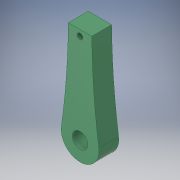
# Autodesk Inventor part: joint3_rot
Saved by Autodesk Inventor 2019 (Build 230136000, 136)
## iProperties
Created: 2019-12-29
Part Number: joint3_rot
Material: Пластик АБС
Document SubType Name: Modeling
Designer: Петров Иван
Density: 1.06 g/cm^3
Appearance: Гладкий — темный цвет морской волны
Author: Петров Иван
Autodesk Inventor part; units mm, degrees
ref_plane "YZ Plane" through (0, 0, 0) normal (1, 0, 0) x (0, 1, 0)
ref_plane "XZ Plane" through (0, 0, 0) normal (0, 1, 0) x (-1, 0, 0)
ref_plane "XY Plane" through (0, 0, 0) normal (0, 0, 1) x (1, 0, 0)
sketch "Эскиз1" plane through (0, 0, 0) normal (0, 0, 1) x (1, 0, 0)
  circle A0 centre (0, 0) radius 3.9
  line L0 (-3.9, 0) -> (-3.9, 42.3207)
  line L1 (3.9, 42.3207) -> (3.9, 0)
  arc A1 (3.9, 42.3207) -> (-3.9, 42.3207) centre (0, 0) ccw
  line L2 (-3.9, 42.3207) -> (-3.9, 48.3207)
  line L3 (-3.9, 48.3207) -> (3.9, 48.3207)
  line L4 (3.9, 48.3207) -> (3.9, 42.3207)
  circle A2 centre (0, 0) radius 7.5
  point P0 (0, 0)
  point P1 (0, -39)
  dimension "d0" = 0
  dimension "d1" = 6
  dimension "d2" = 15
  constraints: 10 end point, 4 point on circle, 3 centre point, 2 perpendicular, 2 vertical, 1 coincident, 1 parallel, 1 tangent
  measures "d0" distance of A0.centre A1.centre
  measures "d1" distance of L0.end L2.end
  measures "d2" diameter of A2
extrude "Выдавливание1" add sketch "Эскиз1" along normal blind 10 contours L1 A2 L0 A0 | A0 L0 A2 L1 | A2 L0 A1 L1 | A1 L2 L3 L4
sketch "Эскиз2" plane through (0, 0, 10) normal (0, 0, 1) x (1, 0, 0)
  line L0 (3.9, 48.3207) -> (-3.9, 48.3207) projected
  line L1 (0, 48.3207) -> (0, 45.3207)
  circle A0 centre (0, 45.3207) radius 1.4
  point P0 (0, 0)
  dimension "d6" = 3
  dimension "d7" = 2.8
  constraints: 2 end point, 1 centre point, 1 coincident, 1 midpoint, 1 vertical
  measures "d6" distance of L1.start L1.end
  measures "d7" diameter of A0
extrude "Выдавливание2" cut sketch "Эскиз2" against normal blind 57.25
thicken "Толщина1" operation add thickness 2 both sides no extend neighbours yes toward (1, 0, 0) faces at (3.9, 20.3777, 3.3333) (-4.4139, 6.0636, 3.3333) (-3.9, 34.3492, 3.3333)
fillet "Сопряжение2" radius 354.75 2 edges at (5.9, 7.4458, 5) (-5.9, 7.4458, 5)
